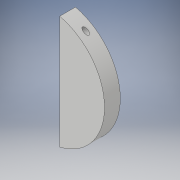
# Autodesk Inventor part: Contrapeso4
Saved by Autodesk Inventor 2019 (Build 230136000, 136)
## iProperties
Created: 2019-06-29
Part Number: Contrapeso4
Material: Generic
Document SubType Name: Modeling
Designer: usuario
Density: 1 g/cm^3
Appearance: Default
Author: usuario
Autodesk Inventor part; units mm, degrees
ref_plane "YZ Plane" through (0, 0, 0) normal (1, 0, 0) x (0, 1, 0)
ref_plane "XZ Plane" through (0, 0, 0) normal (0, 1, 0) x (-1, 0, 0)
ref_plane "XY Plane" through (0, 0, 0) normal (0, 0, 1) x (1, 0, 0)
sketch "Sketch1" plane through (0, 0, 0) normal (0, 0, 1) x (1, 0, 0)
  line L0 (6.2115, -26.7893) -> (6.2115, 26.924)
  line L1 (6.2115, 26.7893) -> (6.2115, -26.7893)
  arc A0 (6.2115, -26.924) -> (6.2115, 26.924) centre (-0.1699, 0) ccw
  line L2 (6.2115, 26.924) -> (6.2115, -26.924)
  point P0 (0, 0)
  point P1 (-5.2115, 24.6247)
  constraints: 6 end point, 2 point on circle, 2 point on line, 1 centre point, 1 collinear
extrude "Extrusion1" add sketch "Sketch1" along normal blind 7.5
sketch "Sketch2" plane through (6.2115, -26.924, 0) normal (-1, 0, 0) x (0, 0, 1)
  line L0 (0, 6.9167) -> (7.5, 6.9167)
  line L1 (0, 0) -> (0, 6.9167)
  line L2 (0, 6.9167) -> (7.5, 6.9167)
  line L3 (7.5, 26.7893) -> (7.5, 0)
  line L4 (7.5, 6.9167) -> (7.5, 0)
  line L5 (7.5, 0) -> (0, 0)
  line L6 (7.5, 0) -> (0, 0)
  circle A0 centre (3.75, 3.4583) radius 1
  line L7 (0, 0) -> (3.0149, 2.7804)
  line L8 (4.4851, 4.1363) -> (7.5, 6.9167)
  line L9 (0, 6.9167) -> (3.0149, 4.1363)
  line L10 (4.4851, 2.7804) -> (7.5, 0)
  line L11 (0, 0) -> (0, 53.5786)
  line L12 (0, 53.5786) -> (0, 0)
  line L13 (0, 26.7893) -> (7.5, 26.7893)
  circle A1 centre (3.75, 50.1203) radius 1
  point P0 (0, 26.924)
  point P1 (280.32, 51.414)
  dimension "d2" = 2
  constraints: 28 end point, 4 point on circle, 2 centre point, 2 perpendicular, 2 vertical, 1 collinear, 1 midpoint, 1 symmetric about line, 1 other
  measures "d2" diameter of A0
extrude "Extrusion2" cut sketch "Sketch2" against normal blind 25.4 contours A0 | A1
body "Solid1"
